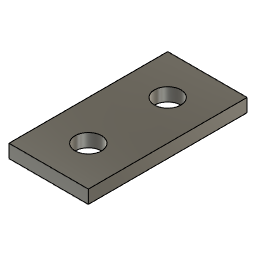
Base+1 (Autodesk Fusion 360 design; units mm, degrees)
Autodesk Fusion 360 part; units mm, degrees
sketch "Esboço3" plane through (0, 0, 0) normal (0, 0, 1) x (1, 0, 0)
box "Primitiva de caixa2" add length 60 width 30 height 5 placed x (0, 1, 0) y (-1, 0, 0) z (0, 0, 1) at (30, 0, 0)
cylinder "Cilindro primitivo2" cut diameter 10 height -35 placed x (1, 0, 0) y (0, 1, 0) z (0, 0, 1) at (15, 15, 5)
cylinder "Cilindro primitivo3" cut diameter 10 height -8 placed x (1, 0, 0) y (0, 1, 0) z (0, 0, 1) at (15, 45, 5)
